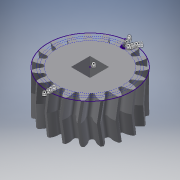
# Autodesk Inventor part: gear 1 shaft herring
Saved by Autodesk Inventor 2017 (Build 210142000, 142)
## iProperties
Created: 2018-04-17
Part Number: gear 1 shaft herring
Material: Generic
Document SubType Name: Modeling
Designer: RKL
Density: 1 g/cm^3
Appearance: Default
Author: RKL
Autodesk Inventor part; units mm, degrees
ref_plane "YZ Plane" through (0, 0, 0) normal (1, 0, 0) x (0, 1, 0)
ref_plane "XZ Plane" through (0, 0, 0) normal (0, 1, 0) x (-1, 0, 0)
ref_plane "XY Plane" through (0, 0, 0) normal (0, 0, 1) x (1, 0, 0)
sketch "Sketch1" plane through (0, 0, 0) normal (0, 0, 1) x (1, 0, 0)
  spline S0 degree 3 poles (-2.891018, 20.800048) (-2.713661, 20.576676) (-2.358963, 20.129952) (-1.902628, 19.404353) (-1.589456, 18.763115) (-1.389993, 18.227388) (-1.335894, 17.947166) (-1.308858, 17.807127) knots 0 0 0 0 0.25006204 0.50010057 0.75007214 0.87510025 1 1 1 1
  spline S1 degree 3 poles (-1.308858, 17.807127) (-1.289736, 17.612471) (-1.261048, 17.320446) (-1.139666, 16.948284) (-1.007917, 16.68564) (-0.82026, 16.457559) (-0.578775, 16.286846) (-0.29354, 16.197424) (0, 16.212724) (0.29354, 16.197424) (0.578775, 16.286846) (0.82026, 16.457559) (1.007917, 16.68564) (1.139666, 16.948284) (1.261048, 17.320446) (1.289736, 17.612471) (1.308858, 17.807127) knots 0 0 0 0 0.12499927 0.18752599 0.25006993 0.31255958 0.37503363 0.4374368 0.5 0.5625632 0.62496637 0.68744042 0.74993007 0.81247401 0.87500073 1 1 1 1
  spline S2 degree 3 poles (1.308858, 17.807127) (1.335894, 17.947166) (1.389993, 18.227388) (1.589456, 18.763115) (1.902628, 19.404353) (2.358963, 20.129952) (2.713661, 20.576676) (2.891018, 20.800048) knots 0 0 0 0 0.12489975 0.24992786 0.49989943 0.74993796 1 1 1 1
  circle A0 centre (0, 0) radius 16.20762 construction
  circle A1 centre (0, 0) radius 17.85416 construction
  circle A2 centre (0, 0) radius 19 construction
  circle A3 centre (0, 0) radius 21
  point P0 (-2.371558, 20.120665)
  point P1 (-1.916009, 19.396968)
  point P2 (-1.543856, 18.62731)
  point P3 (-1.40136, 18.224152)
  point P4 (-1.223794, 17.228911)
  point P5 (-1.13289, 16.951058)
  point P6 (-0.998544, 16.691319)
  point P7 (-0.811243, 16.467079)
  point P8 (-0.571404, 16.300348)
  point P9 (-0.292426, 16.214909)
  point P10 (0, 16.20762)
  point P11 (0.292426, 16.214909)
  point P12 (0.571404, 16.300348)
  point P13 (0.811243, 16.467079)
  point P14 (0.998544, 16.691319)
  point P15 (1.13289, 16.951058)
  point P16 (1.223794, 17.228911)
  point P17 (1.40136, 18.224152)
  point P18 (1.543856, 18.62731)
  point P19 (1.916009, 19.396968)
  point P20 (2.371558, 20.120665)
  constraints: 4 centre point, 2 point on circle, 57 other
extrude "Extrusion1" add sketch "Sketch1" against normal blind 20
extrude "Extrusion2" [suppressed]
pattern_circular "Circular Pattern1" [suppressed]
sketch "Sketch2" plane through (0, 0, 0) normal (0, 0, 1) x (1, 0, 0)
  line L0 (4.7625, -4.7625) -> (-4.7625, -4.7625)
  line L1 (-4.7625, -4.7625) -> (-4.7625, 4.7625)
  line L2 (-4.7625, 4.7625) -> (4.7625, 4.7625)
  line L3 (4.7625, 4.7625) -> (4.7625, -4.7625)
  line L4 (4.7625, -4.7625) -> (-4.7625, 4.7625) construction
  line L5 (-4.7625, -4.7625) -> (4.7625, 4.7625) construction
  point P0 (0, 0)
  dimension "d7" = 9.525
  constraints: 12 end point, 2 midpoint, 2 parallel, 2 perpendicular, 1 horizontal
  measures "d7" distance of L0.end L1.end
extrude "Extrusion3" cut sketch "Sketch2" against normal through all
coil "Coil1" sketch "Sketch1" operation cut axis through (0, 0, -10) along (0, 0, -1) pitch 1000 turns 0.01 hand right contours A3 S2 S1 S0
sketch "Sketch3" plane through (0, 0, -10) normal (0, 0, 1) x (0.9980267, -0.0627905, 0)
  spline S0 degree 3 poles (-1.308858, 17.807127) (-1.335894, 17.947166) (-1.389993, 18.227388) (-1.589456, 18.763115) (-1.902628, 19.404353) (-2.358963, 20.129952) (-2.713661, 20.576676) (-2.891018, 20.800048) knots 0 0 0 0 0.12489975 0.24992786 0.49989943 0.74993796 1 1 1 1
  spline S1 degree 3 poles (1.308858, 17.807127) (1.289736, 17.612471) (1.261048, 17.320446) (1.139666, 16.948284) (1.007917, 16.68564) (0.82026, 16.457559) (0.578775, 16.286846) (0.29354, 16.197424) (0, 16.212724) (-0.29354, 16.197424) (-0.578775, 16.286846) (-0.82026, 16.457559) (-1.007917, 16.68564) (-1.139666, 16.948284) (-1.261048, 17.320446) (-1.289736, 17.612471) (-1.308858, 17.807127) knots 0 0 0 0 0.12499927 0.18752599 0.25006993 0.31255958 0.37503363 0.4374368 0.5 0.5625632 0.62496637 0.68744042 0.74993007 0.81247401 0.87500073 1 1 1 1
  spline S2 degree 3 poles (2.891018, 20.800048) (2.713661, 20.576676) (2.358963, 20.129952) (1.902628, 19.404353) (1.589456, 18.763115) (1.389993, 18.227388) (1.335894, 17.947166) (1.308858, 17.807127) knots 0 0 0 0 0.25006204 0.50010057 0.75007214 0.87510025 1 1 1 1
  arc A0 (2.891018, 20.800048) -> (-2.891018, 20.800048) centre (0, 0) ccw
  constraints: 1 horizontal alignment, 2 other
coil "Coil2" sketch "Sketch3" operation cut axis through (0, 0, -10) along (0, 0, -1) pitch 1000 turns 0.01 hand left
pattern_circular "Circular Pattern2" count 19 over 360 about axis through (0, 0, 0) along (0, 0, -1) of "Coil1", "Coil2"
equation "\"d0\" = FaceWidth"
equation "\"Module\" = 2"
equation "\"PressureAngle\" = 20deg"
equation "\"UnitProfileClearance\" = 0.25"
equation "\"UnitRoundRadius\" = 0.3335"
equation "\"HeadDiameter\" = 42"
equation "\"RootDiameter\" = 32.41524"
equation "\"BaseDiameter\" = 35.70832"
equation "\"PitchDiameter\" = 38"
equation "\"FaceWidth\" = 20"
equation "\"HelixAngle\" = 0"
equation "\"UnitCorrection\" = 0"
equation "\"UnitAddendumModification\" = 0"
equation "\"CircularPitch\" = 6.283185"
equation "\"UnitBacklashShift\" = -0.14619"
equation "\"TotalToolShift\" = -0.29238"
equation "\"IsInternal\" = 0"
body "Solid1"
